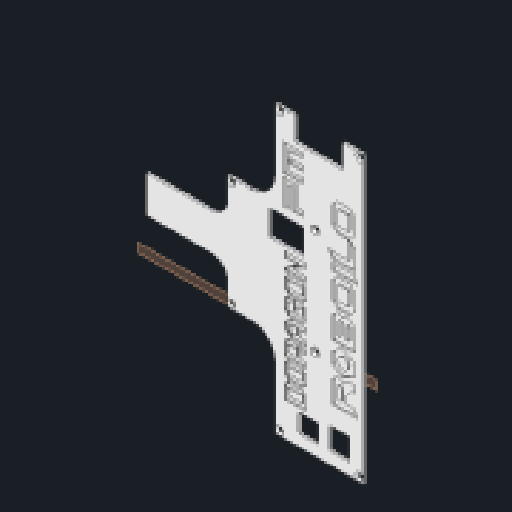
# Autodesk Inventor part: ceil
Saved by Autodesk Inventor 2023 (Build 270158000, 158)
## iProperties
Created: 2024-05-26
Part Number: ceil
Material: ABS Plastic
Document SubType Name: Modeling
Designer: szymo
Density: 1.06 g/cm^3
Appearance: Smooth - White
Mass: 19.1386 g
Surface Area: 254.518 cm^2
Volume: 18.0553 cm^3
TOTAL MASS: 0.0
Author: szymo
Autodesk Inventor part; units mm, degrees
ref_plane "YZ Plane" through (0, 0, 0) normal (1, 0, 0) x (0, 1, 0)
ref_plane "XZ Plane" through (0, 0, 0) normal (0, 1, 0) x (-1, 0, 0)
ref_plane "XY Plane" through (0, 0, 0) normal (0, 0, 1) x (1, 0, 0)
ref_plane "Work Plane1" through (-50.5, 0, 0) normal (0, 0, 1) x (1, 0, 0)
sketch "Sketch3" plane through (-50.5, 0, 0) normal (0, 0, 1) x (1, 0, 0)
  line L0 (0, 0) -> (135.5648, 0) projected
  line L1 (135.5648, 0) -> (135.5648, 5) projected
  line L2 (0, 5) -> (135.5648, 5) projected
  line L3 (0, 0) -> (0, 5) projected
  line L4 (0, 24) -> (50.5, 24) projected
  line L5 (0, 47) -> (50.5, 47) projected
  line L6 (0, 71) -> (135.5648, 71) projected
  line L7 (0, 71) -> (0, 66) projected
  line L8 (0, 66) -> (135.5648, 66) projected
  line L9 (135.5648, 71) -> (135.5648, 66) projected
  arc A0 (130.5648, 120.5) -> (131.5648, 119.5) centre (131.5648, 120.5) ccw projected
  line L10 (131.5648, 119.5) -> (134.5648, 119.5) projected
  arc A1 (134.5648, 119.5) -> (135.5648, 120.5) centre (134.5648, 120.5) ccw projected
  line L11 (135.5648, 124.5) -> (135.5648, 120.5) projected
  line L12 (135.5648, 124.5) -> (51.5, 124.5) projected
  line L13 (51.5, 123.5) -> (80.5, 123.5) projected
  line L14 (80.5, 123.5) -> (80.5, 120.5) projected
  arc A2 (80.5, 120.5) -> (81.5, 119.5) centre (81.5, 120.5) ccw projected
  line L15 (81.5, 119.5) -> (84.5, 119.5) projected
  arc A3 (84.5, 119.5) -> (85.5, 120.5) centre (84.5, 120.5) ccw projected
  line L16 (85.5, 123.5) -> (85.5, 120.5) projected
  line L17 (85.5, 123.5) -> (130.5648, 123.5) projected
  line L18 (130.5648, 123.5) -> (130.5648, 120.5) projected
  circle A4 centre (133.0648, 122) radius 1.75 projected
  circle A5 centre (83, 122) radius 1.75 projected
  line L19 (120.8148, 112) -> (120.8148, 123) projected
  line L20 (120.8148, 123) -> (94.8148, 123) projected
  line L21 (94.8148, 123) -> (94.8148, 112) projected
  line L22 (94.8148, 112) -> (120.8148, 112) projected
  arc A6 (131.5648, -48.5) -> (130.5648, -49.5) centre (131.5648, -49.5) ccw projected
  line L23 (130.5648, -52.5) -> (130.5648, -49.5) projected
  line L24 (85.5, -52.5) -> (130.5648, -52.5) projected
  line L25 (85.5, -52.5) -> (85.5, -49.5) projected
  arc A7 (85.5, -49.5) -> (84.5, -48.5) centre (84.5, -49.5) ccw projected
  line L26 (81.5, -48.5) -> (84.5, -48.5) projected
  arc A8 (81.5, -48.5) -> (80.5, -49.5) centre (81.5, -49.5) ccw projected
  line L27 (80.5, -52.5) -> (80.5, -49.5) projected
  line L28 (51.5, -52.5) -> (80.5, -52.5) projected
  line L29 (135.5648, -53.5) -> (51.5, -53.5) projected
  line L30 (135.5648, -53.5) -> (135.5648, -49.5) projected
  arc A9 (135.5648, -49.5) -> (134.5648, -48.5) centre (134.5648, -49.5) ccw projected
  line L31 (131.5648, -48.5) -> (134.5648, -48.5) projected
  circle A10 centre (133.0648, -51) radius 1.75 projected
  circle A11 centre (83, -51) radius 1.75 projected
  line L32 (95.5648, -45.8) -> (95.5648, -35.2) projected
  line L33 (106.8648, -35.2) -> (95.5648, -35.2) projected
  line L34 (106.8648, -35.2) -> (106.8648, -45.8) projected
  line L35 (95.5648, -45.8) -> (106.8648, -45.8) projected
  circle A12 centre (90.4898, -49.075) radius 1.675 projected
  circle A13 centre (124.5398, -49.075) radius 1.675 projected
  line L36 (126.3648, -33.5) -> (126.3648, -45.5) projected
  line L37 (126.3648, -45.5) -> (114.7648, -45.5) projected
  line L38 (114.7648, -45.5) -> (114.7648, -33.5) projected
  line L39 (114.7648, -33.5) -> (86.8648, -33.5) projected
  line L40 (86.8648, -33.5) -> (86.8648, -52.5) projected
  line L41 (86.8648, -52.5) -> (128.0648, -52.5) projected
  line L42 (128.0648, -52.5) -> (128.0648, -33.5) projected
  line L43 (128.0648, -33.5) -> (126.3648, -33.5) projected
  line L44 (126.3648, -32.7) -> (114.7648, -32.7) projected
  line L45 (114.7648, -32.7) -> (114.7648, -45.5) projected
  line L46 (114.7648, -45.5) -> (126.3648, -45.5) projected
  line L47 (126.3648, -45.5) -> (126.3648, -32.7) projected
  line L48 (80.5, -53.5) -> (135.5648, -53.5)
  line L49 (135.5648, -53.5) -> (135.5648, 124.5)
  line L50 (135.5648, 124.5) -> (80.5, 124.5)
  line L51 (80.5, 124.5) -> (80.5, -53.5)
  line L52 (0, 24) -> (80.5, 24)
  line L53 (80.5, 24) -> (80.5, 47)
  line L54 (80.5, 47) -> (0, 47)
  line L55 (0, 47) -> (0, 24)
  line L56 (80.5, 24) -> (50.5, 24)
  line L57 (50.5, 24) -> (50.5, 0)
  line L58 (50.5, 0) -> (80.5, 0)
  line L59 (80.5, 0) -> (80.5, 24)
  line L60 (50.5, 47) -> (80.5, 47)
  line L61 (80.5, 47) -> (80.5, 71)
  line L62 (80.5, 71) -> (50.5, 71)
  line L63 (50.5, 71) -> (50.5, 47)
  arc A14 (97.9124, 51.3) -> (98.0124, 51.4) centre (97.9124, 51.4) ccw projected
  line L64 (77.4124, 51.3) -> (97.9124, 51.3) projected
  arc A15 (77.3124, 51.4) -> (77.4124, 51.3) centre (77.4124, 51.4) ccw projected
  line L65 (77.3124, 65.9) -> (77.3124, 51.4) projected
  arc A16 (77.4124, 66) -> (77.3124, 65.9) centre (77.4124, 65.9) ccw projected
  line L66 (97.9124, 66) -> (77.4124, 66) projected
  arc A17 (98.0124, 65.9) -> (97.9124, 66) centre (97.9124, 65.9) ccw projected
  line L67 (98.0124, 51.4) -> (98.0124, 65.9) projected
  line L68 (96.2124, 64.1) -> (96.2124, 53.2) projected
  arc A18 (96.2124, 64.1) -> (95.9124, 64.4) centre (95.9124, 64.1) ccw projected
  line L69 (95.9124, 64.4) -> (95.8124, 64.4) projected
  line L70 (95.8124, 64.4) -> (95.3509, 64.95) projected
  line L71 (95.3509, 64.95) -> (94.9739, 64.95) projected
  line L72 (94.9739, 64.95) -> (94.5124, 64.4) projected
  line L73 (94.5124, 64.4) -> (90.8124, 64.4) projected
  line L74 (90.8124, 64.4) -> (90.8124, 64.75) projected
  line L75 (90.8124, 64.75) -> (89.5124, 64.75) projected
  line L76 (89.5124, 64.4) -> (89.5124, 64.75) projected
  line L77 (89.5124, 64.4) -> (85.8124, 64.4) projected
  line L78 (85.8124, 64.4) -> (85.8124, 64.75) projected
  line L79 (85.8124, 64.75) -> (84.5124, 64.75) projected
  line L80 (84.5124, 64.4) -> (84.5124, 64.75) projected
  line L81 (84.5124, 64.4) -> (80.8124, 64.4) projected
  line L82 (80.8124, 64.4) -> (80.3509, 64.95) projected
  line L83 (80.3509, 64.95) -> (79.9739, 64.95) projected
  line L84 (79.9739, 64.95) -> (79.5124, 64.4) projected
  line L85 (79.5124, 64.4) -> (79.4124, 64.4) projected
  arc A19 (79.4124, 64.4) -> (79.1124, 64.1) centre (79.4124, 64.1) ccw projected
  line L86 (79.1124, 64.1) -> (79.1124, 53.2) projected
  arc A20 (79.1124, 53.2) -> (79.4124, 52.9) centre (79.4124, 53.2) ccw projected
  line L87 (79.4124, 52.9) -> (79.5124, 52.9) projected
  line L88 (79.5124, 52.9) -> (79.9739, 52.35) projected
  line L89 (80.3509, 52.35) -> (79.9739, 52.35) projected
  line L90 (80.3509, 52.35) -> (80.8124, 52.9) projected
  line L91 (80.8124, 52.9) -> (84.5124, 52.9) projected
  line L92 (84.5124, 52.9) -> (84.5124, 52.55) projected
  line L93 (85.8124, 52.55) -> (84.5124, 52.55) projected
  line L94 (85.8124, 52.9) -> (85.8124, 52.55) projected
  line L95 (85.8124, 52.9) -> (89.5124, 52.9) projected
  line L96 (89.5124, 52.9) -> (89.5124, 52.55) projected
  line L97 (90.8124, 52.55) -> (89.5124, 52.55) projected
  line L98 (90.8124, 52.9) -> (90.8124, 52.55) projected
  line L99 (90.8124, 52.9) -> (94.5124, 52.9) projected
  line L100 (94.5124, 52.9) -> (94.9739, 52.35) projected
  line L101 (95.3509, 52.35) -> (94.9739, 52.35) projected
  line L102 (95.3509, 52.35) -> (95.8124, 52.9) projected
  line L103 (95.8124, 52.9) -> (95.9124, 52.9) projected
  arc A21 (95.9124, 52.9) -> (96.2124, 53.2) centre (95.9124, 53.2) ccw projected
  line L104 (78.1624, 55.75) -> (78.8624, 55.75) projected
  line L105 (78.8624, 55.75) -> (78.8624, 61.55) projected
  line L106 (78.1624, 61.55) -> (78.8624, 61.55) projected
  line L107 (78.1624, 61.55) -> (78.1624, 55.75) projected
  line L108 (97.1624, 61.55) -> (97.1624, 55.75) projected
  line L109 (96.4624, 61.55) -> (97.1624, 61.55) projected
  line L110 (96.4624, 55.75) -> (96.4624, 61.55) projected
  line L111 (96.4624, 55.75) -> (97.1624, 55.75) projected
  arc A22 (76.8124, 51.4) -> (77.4124, 50.8) centre (77.4124, 51.4) ccw
  line L112 (77.4124, 50.8) -> (97.9124, 50.8)
  arc A23 (97.9124, 50.8) -> (98.5124, 51.4) centre (97.9124, 51.4) ccw
  line L113 (98.5124, 51.4) -> (98.5124, 65.9)
  arc A24 (98.5124, 65.9) -> (97.9124, 66.5) centre (97.9124, 65.9) ccw
  line L114 (97.9124, 66.5) -> (77.4124, 66.5)
  arc A25 (77.4124, 66.5) -> (76.8124, 65.9) centre (77.4124, 65.9) ccw
  line L115 (76.8124, 65.9) -> (76.8124, 51.4)
  line L116 (95.0648, -34.7) -> (95.0648, -46.3)
  line L117 (95.0648, -46.3) -> (107.3648, -46.3)
  line L118 (107.3648, -46.3) -> (107.3648, -34.7)
  line L119 (107.3648, -34.7) -> (95.0648, -34.7)
  line L120 (114.2648, -45.5) -> (114.2648, -32.2)
  line L121 (114.2648, -32.2) -> (126.8648, -32.2)
  line L122 (126.8648, -32.2) -> (126.8648, -45.5)
  line L123 (126.3648, -46) -> (114.7648, -46)
  line L124 (92.8148, 110) -> (92.8148, 125)
  line L125 (92.8148, 125) -> (122.8148, 125)
  line L126 (122.8148, 125) -> (122.8148, 110)
  line L127 (122.8148, 110) -> (92.8148, 110)
  line L128 (114.2648, -45.5) -> (114.2648, -46)
  line L129 (114.2648, -46) -> (114.7648, -46)
  line L130 (126.3648, -46) -> (126.8648, -46)
  line L131 (126.8648, -46) -> (126.8648, -45.5)
  line L132 (51.5, -53.5) -> (51.5, -52.5) projected
  line L133 (51.5, 124.5) -> (51.5, 123.5) projected
  circle A26 centre (105.3205, 68.5) radius 1.75 projected
  circle A27 centre (53, 68.5) radius 1.75 projected
  line L134 (0, 47) -> (0, 42.5) projected
  line L135 (0, 42.5) -> (50.5, 42.5) projected
  line L136 (50.5, 47) -> (50.5, 42.5) projected
  line L137 (50.5, 24) -> (50.5, 28.5) projected
  line L138 (0, 28.5) -> (50.5, 28.5) projected
  line L139 (0, 24) -> (0, 28.5) projected
  circle A28 centre (105.3205, 2.5) radius 1.75 projected
  circle A29 centre (53, 2.5) radius 1.75 projected
  point P0 (122.8148, 124.5)
  point P1 (92.8148, 124.5)
  point P2 (80.5, 0)
  point P3 (0, 44)
  point P4 (50.5, 44)
  point P5 (122.8148, 124.5)
  point P6 (122.8148, 123.5)
  point P7 (92.8148, 123.5)
  point P8 (92.8148, 124.5)
  point P9 (50.5, 66)
  point P10 (50.5, 5)
  point P11 (80.5, 66)
  point P12 (80.5, 5)
  point P13 (50.5, 27)
  point P14 (0, 27)
  dimension "d16" = 0.5
  dimension "d17" = 0.5
  dimension "d18" = 0.5
  dimension "d19" = 0.5
  dimension "d20" = 2
  constraints: 72 end point, 9 parallel, 8 point on circle, 6 perpendicular, 5 point on line, 4 centre point, 4 horizontal, 2 collinear, 1 vertical, 15 other
  measures "d16" distance between parallel lines of L65 L115
  measures "d17" distance between parallel lines of L32 L116
  measures "d18" distance between parallel lines of L45 L120
  measures "d19" distance between parallel lines of L37 L123
  measures "d20" distance between parallel lines of L21 L124
extrude "Extrusion2" add sketch "Sketch3" along normal blind 1.5 contours L57 L2 L51 L0 | L51 L2 L1 L0 | L0 L49 A9 L31 A6 L23 L24 L42 L43 L122 L121 L120 L39 L40 L25 A7 L26 A8 L51 | L57 L52 L51 L2 | A8 L26 A7 L25 L24 L23 A6 L31 A9 L30 L29 L51 L27 | L51 L112 A23 L113 A24 L8 L49 L2 | L137 L138 L55 L135 L136 L54 L51 L52 | L4 L55 L138 L137 | L8 A24 L114 L51 L6 L9 | L54 L63 L8 A25 L115 A22 L112 L51 | L6 L51 A2 L15 A3 L16 L17 L124 L127 L126 L18 A0 L10 A1 L49 | L136 L135 L55 L5 | L51 L114 A25 L8 L63 L6 | A1 L10 A0 L18 L17 L126 L12 L11 | L14 L51 L12 L124 L17 L16 A3 L15 A2 | L40 L39 L120 L128 L129 L123 L130 L131 L122 L43 L42 L24 | A4 | A5 | A10 | A11 | A12 | A13 | A26 | A27 | A28 | A29
fillet "Fillet2" radius 1 10 edges at (44.5648, -46.3, 0.75) (44.5648, -34.7, 0.75) (56.8648, -34.7, 0.75) (56.8648, -46.3, 0.75) (63.7648, -46, 0.75) (63.7648, -32.2, 0.75) (76.3648, -32.2, 0.75) (76.3648, -46, 0.75) (42.3148, 110, 0.75) (72.3148, 110, 0.75)
fillet "Fillet3" radius 15 2 edges at (30, 0, 0.75) (30, 71, 0.75)
sketch "Sketch4" plane through (-50.5, 0, 1.5) normal (0, 0, 1) x (1, 0, 0)
  arc A0 (131.5648, -48.5) -> (130.5648, -49.5) centre (131.5648, -49.5) ccw projected
  line L0 (130.5648, -52.5) -> (130.5648, -49.5) projected
  line L1 (85.5, -52.5) -> (130.5648, -52.5) projected
  line L2 (85.5, -52.5) -> (85.5, -49.5) projected
  arc A1 (85.5, -49.5) -> (84.5, -48.5) centre (84.5, -49.5) ccw projected
  line L3 (81.5, -48.5) -> (84.5, -48.5) projected
  arc A2 (81.5, -48.5) -> (80.5, -49.5) centre (81.5, -49.5) ccw projected
  line L4 (80.5, -52.5) -> (80.5, -49.5) projected
  line L5 (51.5, -52.5) -> (80.5, -52.5) projected
  line L6 (135.5648, -53.5) -> (51.5, -53.5) projected
  line L7 (135.5648, -53.5) -> (135.5648, -49.5) projected
  arc A3 (135.5648, -49.5) -> (134.5648, -48.5) centre (134.5648, -49.5) ccw projected
  line L8 (131.5648, -48.5) -> (134.5648, -48.5) projected
  circle A4 centre (133.0648, -51) radius 1.75 projected
  circle A5 centre (83, -51) radius 1.75 projected
  arc A6 (130.5648, 120.5) -> (131.5648, 119.5) centre (131.5648, 120.5) ccw projected
  line L9 (131.5648, 119.5) -> (134.5648, 119.5) projected
  arc A7 (134.5648, 119.5) -> (135.5648, 120.5) centre (134.5648, 120.5) ccw projected
  line L10 (135.5648, 124.5) -> (135.5648, 120.5) projected
  line L11 (135.5648, 124.5) -> (51.5, 124.5) projected
  line L12 (51.5, 123.5) -> (80.5, 123.5) projected
  line L13 (80.5, 123.5) -> (80.5, 120.5) projected
  arc A8 (80.5, 120.5) -> (81.5, 119.5) centre (81.5, 120.5) ccw projected
  line L14 (81.5, 119.5) -> (84.5, 119.5) projected
  arc A9 (84.5, 119.5) -> (85.5, 120.5) centre (84.5, 120.5) ccw projected
  line L15 (85.5, 123.5) -> (85.5, 120.5) projected
  line L16 (85.5, 123.5) -> (130.5648, 123.5) projected
  line L17 (130.5648, 123.5) -> (130.5648, 120.5) projected
  circle A10 centre (133.0648, 122) radius 1.75 projected
  circle A11 centre (83, 122) radius 1.75 projected
  line L18 (0, 71) -> (135.5648, 71) projected
  line L19 (0, 71) -> (0, 66) projected
  line L20 (0, 66) -> (135.5648, 66) projected
  line L21 (135.5648, 71) -> (135.5648, 66) projected
  line L22 (0, 0) -> (135.5648, 0) projected
  line L23 (135.5648, 0) -> (135.5648, 5) projected
  line L24 (0, 5) -> (135.5648, 5) projected
  line L25 (0, 0) -> (0, 5) projected
  line L26 (0, 24) -> (50.5, 24) projected
  line L27 (0, 47) -> (50.5, 47) projected
  line L28 (51.5, 124.5) -> (51.5, 123.5) projected
  line L29 (51.5, -53.5) -> (51.5, -52.5) projected
  circle A12 centre (105.3205, 68.5) radius 1.75 projected
  circle A13 centre (53, 68.5) radius 1.75 projected
  line L30 (0, 47) -> (0, 42.5) projected
  line L31 (0, 42.5) -> (50.5, 42.5) projected
  line L32 (50.5, 47) -> (50.5, 42.5) projected
  line L33 (50.5, 24) -> (50.5, 28.5) projected
  line L34 (0, 28.5) -> (50.5, 28.5) projected
  line L35 (0, 24) -> (0, 28.5) projected
  circle A14 centre (105.3205, 2.5) radius 1.75 projected
  circle A15 centre (53, 2.5) radius 1.75 projected
  point P0 (50.5, 0)
  point P1 (0, 44)
  point P2 (50.5, 44)
  point P3 (50.5, 27)
  point P4 (0, 27)
  constraints: 8 coincident
hole "Hole2" at (32.5, -51, 1.5) at (82.5648, -51, 1.5) at (82.5648, 122, 1.5) at (32.5, 122, 1.5) at (54.8205, 68.5, 1.5) at (54.8205, 2.5, 1.5) at (2.5, 2.5, 1.5) at (2.5, 68.5, 1.5) direction (0, 0, -1) diameter 2.9 end through all countersink diameter 5.5 countersink angle 90 clearance for "Countersunk Flat Head Screw ISO 2009/7046" size "M2.5" standard "ISO"
fillet "Fillet4" radius 10 2 edges at (0, 24, 0.75) (0, 47, 0.75)
sketch "Sketch5" plane through (-50.5, 0, 1.5) normal (0, 0, 1) x (1, 0, 0)
  arc A0 (54.1456, 0) -> (50.5, 3.6456) centre (53, 2.5) ccw projected
  line L0 (54.1456, 0) -> (65.5, 0) projected
  arc A1 (80.5, -15) -> (65.5, 0) centre (65.5, -15) ccw projected
  line L1 (80.5, -15) -> (80.5, -49.8544) projected
  arc A2 (84.1456, -53.5) -> (80.5, -49.8544) centre (83, -51) ccw projected
  line L2 (84.1456, -53.5) -> (131.9191, -53.5) projected
  arc A3 (135.5648, -49.8544) -> (131.9191, -53.5) centre (133.0648, -51) ccw projected
  line L3 (135.5648, -49.8544) -> (135.5648, 120.8544) projected
  arc A4 (131.9191, 124.5) -> (135.5648, 120.8544) centre (133.0648, 122) ccw projected
  line L4 (131.9191, 124.5) -> (122.8148, 124.5) projected
  line L5 (122.8148, 124.5) -> (122.8148, 111) projected
  arc A5 (121.8148, 110) -> (122.8148, 111) centre (121.8148, 111) ccw projected
  line L6 (121.8148, 110) -> (93.8148, 110) projected
  arc A6 (92.8148, 111) -> (93.8148, 110) centre (93.8148, 111) ccw projected
  line L7 (92.8148, 111) -> (92.8148, 124.5) projected
  line L8 (92.8148, 124.5) -> (84.1456, 124.5) projected
  arc A7 (80.5, 120.8544) -> (84.1456, 124.5) centre (83, 122) ccw projected
  line L9 (80.5, 120.8544) -> (80.5, 86) projected
  arc A8 (65.5, 71) -> (80.5, 86) centre (65.5, 86) ccw projected
  line L10 (65.5, 71) -> (54.1456, 71) projected
  arc A9 (50.5, 67.3544) -> (54.1456, 71) centre (53, 68.5) ccw projected
  line L11 (50.5, 67.3544) -> (50.5, 57) projected
  arc A10 (40.5, 47) -> (50.5, 57) centre (40.5, 57) ccw projected
  line L12 (40.5, 47) -> (0, 47) projected
  line L13 (0, 47) -> (0, 24) projected
  line L14 (0, 24) -> (40.5, 24) projected
  arc A11 (50.5, 14) -> (40.5, 24) centre (40.5, 14) ccw projected
  line L15 (50.5, 14) -> (50.5, 3.6456) projected
  circle A12 centre (105.3205, 68.5) radius 2.75 projected
  circle A13 centre (105.3205, 2.5) radius 2.75 projected
  line L16 (77.4124, 66.5) -> (97.9124, 66.5) projected
  arc A14 (98.5124, 65.9) -> (97.9124, 66.5) centre (97.9124, 65.9) ccw projected
  line L17 (98.5124, 65.9) -> (98.5124, 51.4) projected
  arc A15 (97.9124, 50.8) -> (98.5124, 51.4) centre (97.9124, 51.4) ccw projected
  line L18 (97.9124, 50.8) -> (77.4124, 50.8) projected
  arc A16 (76.8124, 51.4) -> (77.4124, 50.8) centre (77.4124, 51.4) ccw projected
  line L19 (76.8124, 51.4) -> (76.8124, 65.9) projected
  arc A17 (77.4124, 66.5) -> (76.8124, 65.9) centre (77.4124, 65.9) ccw projected
  line L20 (114.2648, -45) -> (114.2648, -33.2) projected
  arc A18 (115.2648, -32.2) -> (114.2648, -33.2) centre (115.2648, -33.2) ccw projected
  line L21 (115.2648, -32.2) -> (125.8648, -32.2) projected
  arc A19 (126.8648, -33.2) -> (125.8648, -32.2) centre (125.8648, -33.2) ccw projected
  line L22 (126.8648, -33.2) -> (126.8648, -45) projected
  arc A20 (125.8648, -46) -> (126.8648, -45) centre (125.8648, -45) ccw projected
  line L23 (125.8648, -46) -> (115.2648, -46) projected
  arc A21 (114.2648, -45) -> (115.2648, -46) centre (115.2648, -45) ccw projected
  line L24 (96.0648, -34.7) -> (106.3648, -34.7) projected
  arc A22 (107.3648, -35.7) -> (106.3648, -34.7) centre (106.3648, -35.7) ccw projected
  line L25 (107.3648, -35.7) -> (107.3648, -45.3) projected
  arc A23 (106.3648, -46.3) -> (107.3648, -45.3) centre (106.3648, -45.3) ccw projected
  line L26 (106.3648, -46.3) -> (96.0648, -46.3) projected
  arc A24 (95.0648, -45.3) -> (96.0648, -46.3) centre (96.0648, -45.3) ccw projected
  line L27 (95.0648, -45.3) -> (95.0648, -35.7) projected
  arc A25 (96.0648, -34.7) -> (95.0648, -35.7) centre (96.0648, -35.7) ccw projected
  line L28 (105.3205, -31.7) -> (105.3205, 48.8) construction
  line L29 (105.3205, 48.8) -> (80.5, 48.8) construction
  line L30 (80.5, 48.8) -> (80.5, -31.7) construction
  line L31 (80.5, -31.7) -> (105.3205, -31.7) construction
  line L32 (116.1651, 28.6458) -> (116.1651, 14.5717) projected
  line L33 (125.2148, -10.52) -> (128.2141, -7.4431) projected
  line L34 (128.2141, -7.4431) -> (129.5648, -7.4431) projected
  line L35 (129.5648, -7.4431) -> (129.5648, -3.1151) projected
  line L36 (129.5648, -3.1151) -> (125.5551, -3.1151) projected
  line L37 (125.5551, -3.1151) -> (123.3584, -5.3021) projected
  line L38 (123.3584, -5.3021) -> (120.3535, -3.0659) projected
  line L39 (120.3535, -3.0659) -> (116.1651, -6.1782) projected
  line L40 (116.1651, -6.1782) -> (116.1651, -20.0711) projected
  line L41 (116.1651, -20.0711) -> (131.9602, -20.0711) projected
  line L42 (131.9602, -20.0711) -> (129.4807, -15.7431) projected
  line L43 (129.4807, -15.7431) -> (125.2148, -15.7431) projected
  line L44 (125.2148, -15.7431) -> (125.2148, -10.52) projected
  line L45 (120.6271, -7.6036) -> (121.8612, -8.5098) projected
  line L46 (121.8612, -8.5098) -> (121.8612, -15.7431) projected
  line L47 (121.8612, -15.7431) -> (119.4584, -15.7431) projected
  line L48 (119.4584, -15.7431) -> (119.4584, -8.4973) projected
  line L49 (119.4584, -8.4973) -> (120.6271, -7.6036) projected
  line L50 (129.5648, 1.4254) -> (129.5648, 9.1617) projected
  line L51 (129.5648, 9.1617) -> (122.8649, 13.0299) projected
  line L52 (122.8649, 13.0299) -> (116.1651, 9.1617) projected
  line L53 (116.1651, 9.1617) -> (116.1651, 1.4254) projected
  line L54 (116.1651, 1.4254) -> (122.8649, -2.4427) projected
  line L55 (122.8649, -2.4427) -> (129.5648, 1.4254) projected
  circle A26 centre (122.8649, 5.2936) radius 3.3 projected
  line L56 (129.5848, 14.5717) -> (129.5848, 28.6458) projected
  line L57 (129.5848, 28.6458) -> (125.3867, 31.747) projected
  line L58 (125.3867, 31.747) -> (122.875, 29.8983) projected
  line L59 (122.875, 29.8983) -> (120.3632, 31.747) projected
  line L60 (120.3632, 31.747) -> (116.1651, 28.6458) projected
  line L61 (116.1651, 28.6458) -> (116.1651, 14.5717) projected
  line L62 (116.1651, 14.5717) -> (129.5848, 14.5717) projected
  line L63 (121.3489, 26.1486) -> (121.3489, 18.8997) projected
  line L64 (121.3489, 18.8997) -> (119.4785, 18.8997) projected
  line L65 (119.4785, 18.8997) -> (119.4785, 26.1539) projected
  line L66 (119.4785, 26.1539) -> (120.3691, 26.9374) projected
  line L67 (120.3691, 26.9374) -> (121.3489, 26.1486) projected
  line L68 (124.4011, 18.8997) -> (124.4011, 26.1486) projected
  line L69 (124.4011, 26.1486) -> (125.3808, 26.9374) projected
  line L70 (125.3808, 26.9374) -> (126.2715, 26.1539) projected
  line L71 (126.2715, 26.1539) -> (126.2715, 18.8997) projected
  line L72 (126.2715, 18.8997) -> (124.4011, 18.8997) projected
  line L73 (126.494, 33.3579) -> (129.5648, 36.4286) projected
  line L74 (129.5648, 36.4286) -> (129.5648, 47.4441) projected
  line L75 (129.5648, 47.4441) -> (126.494, 50.5148) projected
  line L76 (126.494, 50.5148) -> (119.2358, 50.5148) projected
  line L77 (119.2358, 50.5148) -> (116.1651, 47.4441) projected
  line L78 (116.1651, 47.4441) -> (116.1651, 36.4286) projected
  line L79 (116.1651, 36.4286) -> (119.2358, 33.3579) projected
  line L80 (119.2358, 33.3579) -> (126.494, 33.3579) projected
  line L81 (126.2715, 37.686) -> (119.4584, 37.686) projected
  line L82 (119.4584, 37.686) -> (119.4584, 46.1868) projected
  line L83 (119.4584, 46.1868) -> (126.2715, 46.1868) projected
  line L84 (126.2715, 46.1868) -> (126.2715, 37.686) projected
  line L85 (131.9586, 52.2145) -> (129.5013, 56.5425) projected
  line L86 (129.5013, 56.5425) -> (116.1651, 56.5425) projected
  line L87 (116.1651, 56.5425) -> (116.1651, 52.2145) projected
  line L88 (116.1651, 52.2145) -> (131.9586, 52.2145) projected
  line L89 (129.5648, 88.0003) -> (126.494, 91.071) projected
  line L90 (126.494, 91.071) -> (119.2358, 91.071) projected
  line L91 (119.2358, 91.071) -> (116.1651, 88.0003) projected
  line L92 (116.1651, 88.0003) -> (116.1651, 76.9848) projected
  line L93 (116.1651, 76.9848) -> (119.2358, 73.9141) projected
  line L94 (119.2358, 73.9141) -> (126.2715, 73.9141) projected
  line L95 (126.2715, 73.9141) -> (126.2715, 62.7008) projected
  line L96 (126.2715, 62.7008) -> (113.738, 62.7008) projected
  line L97 (113.738, 62.7008) -> (116.2396, 58.3727) projected
  line L98 (116.2396, 58.3727) -> (129.5848, 58.3727) projected
  line L99 (129.5848, 58.3727) -> (129.5848, 70.8415) projected
  line L100 (129.5848, 70.8415) -> (126.5032, 73.9232) projected
  line L101 (126.5032, 73.9232) -> (129.5648, 76.9848) projected
  line L102 (129.5648, 76.9848) -> (129.5648, 88.0003) projected
  line L103 (126.2715, 78.2421) -> (119.4584, 78.2421) projected
  line L104 (119.4584, 78.2421) -> (119.4584, 86.743) projected
  line L105 (119.4584, 86.743) -> (126.2715, 86.743) projected
  line L106 (126.2715, 86.743) -> (126.2715, 78.2421) projected
  line L107 (91.5024, 71.975) -> (97.5262, 71.975) projected
  line L108 (97.5262, 71.975) -> (97.5262, 74.9242) projected
  line L109 (97.5262, 74.9242) -> (94.45, 74.9242) projected
  line L110 (94.45, 74.9242) -> (94.45, 87.525) projected
  line L111 (94.45, 87.525) -> (85.5, 87.525) projected
  line L112 (85.5, 87.525) -> (85.5, 71.975) projected
  line L113 (85.5, 71.975) -> (88.675, 71.975) projected
  line L114 (88.675, 71.975) -> (88.675, 84.4887) projected
  line L115 (88.675, 84.4887) -> (91.5024, 84.4887) projected
  line L116 (91.5024, 84.4887) -> (91.5024, 71.975) projected
  line L117 (85.5, 106.5) -> (85.5, 89.825) projected
  line L118 (85.5, 89.825) -> (97.6, 89.825) projected
  line L119 (97.6, 89.825) -> (97.6, 92.775) projected
  line L120 (97.6, 92.775) -> (88.6, 92.775) projected
  line L121 (88.6, 92.775) -> (88.6, 103.4705) projected
  line L122 (88.6, 103.4705) -> (97.5254, 103.4705) projected
  line L123 (97.5254, 103.4705) -> (97.5254, 106.5) projected
  line L124 (97.5254, 106.5) -> (85.5, 106.5) projected
  line L125 (89.7, 99.675) -> (89.7, 96.575) projected
  line L126 (89.7, 96.575) -> (97.6, 96.575) projected
  line L127 (97.6, 96.575) -> (97.6, 99.675) projected
  line L128 (97.6, 99.675) -> (89.7, 99.675) projected
  circle A27 centre (105.3205, 2.5) radius 2.75 projected
  line L129 (99.4102, -32.075) -> (86.4102, -32.075)
  line L130 (86.4102, -32.075) -> (86.4102, -23.2821)
  line L131 (86.4102, -23.2821) -> (88.2317, -23.2821)
  line L132 (88.2317, -23.2821) -> (88.2317, -21.8607)
  line L133 (88.2317, -21.8607) -> (97.5888, -21.8607)
  line L134 (97.5888, -21.8607) -> (97.5888, -23.2821)
  line L135 (97.5888, -23.2821) -> (99.4102, -23.2821)
  line L136 (99.4102, -23.2821) -> (99.4102, -32.075)
  line L137 (97.3317, -24.9679) -> (88.4888, -24.9679)
  line L138 (88.4888, -24.9679) -> (88.4888, -28.9679)
  line L139 (88.4888, -28.9679) -> (97.3317, -28.9679)
  line L140 (97.3317, -28.9679) -> (97.3317, -24.9679)
  line L141 (99.4102, -19.0464) -> (97.5888, -19.0464)
  line L142 (97.5888, -19.0464) -> (97.5888, -20.4679)
  line L143 (97.5888, -20.4679) -> (88.2317, -20.4679)
  line L144 (88.2317, -20.4679) -> (88.2317, -19.0464)
  line L145 (88.2317, -19.0464) -> (86.4102, -19.0464)
  line L146 (86.4102, -19.0464) -> (86.4102, -11.675)
  line L147 (86.4102, -11.675) -> (88.2317, -11.675)
  line L148 (88.2317, -11.675) -> (88.2317, -10.2536)
  line L149 (88.2317, -10.2536) -> (97.5888, -10.2536)
  line L150 (97.5888, -10.2536) -> (97.5888, -11.675)
  line L151 (97.5888, -11.675) -> (99.4102, -11.675)
  line L152 (99.4102, -11.675) -> (99.4102, -19.0464)
  line L153 (97.3317, -13.3607) -> (88.4888, -13.3607)
  line L154 (88.4888, -13.3607) -> (88.4888, -17.3607)
  line L155 (88.4888, -17.3607) -> (97.3317, -17.3607)
  line L156 (97.3317, -17.3607) -> (97.3317, -13.3607)
  line L157 (99.4102, -8.8607) -> (86.4102, -8.8607)
  line L158 (86.4102, -8.8607) -> (86.4102, -0.0679)
  line L159 (86.4102, -0.0679) -> (88.2317, -0.0679)
  line L160 (88.2317, -0.0679) -> (88.2317, 1.3536)
  line L161 (88.2317, 1.3536) -> (93.9531, 1.3536)
  line L162 (93.9531, 1.3536) -> (93.9531, -0.0679)
  line L163 (93.9531, -0.0679) -> (95.5102, -0.0679)
  line L164 (95.5102, -0.0679) -> (95.5102, 1.3536)
  line L165 (95.5102, 1.3536) -> (99.4102, 1.3536)
  line L166 (99.4102, 1.3536) -> (99.4102, -1.7536)
  line L167 (99.4102, -1.7536) -> (95.7674, -1.7536)
  line L168 (95.7674, -1.7536) -> (95.7674, -5.7536)
  line L169 (95.7674, -5.7536) -> (99.4102, -5.7536)
  line L170 (99.4102, -5.7536) -> (99.4102, -8.8607)
  line L171 (93.6959, -1.7536) -> (88.4888, -1.7536)
  line L172 (88.4888, -1.7536) -> (88.4888, -5.7536)
  line L173 (88.4888, -5.7536) -> (93.6959, -5.7536)
  line L174 (93.6959, -5.7536) -> (93.6959, -1.7536)
  line L175 (99.4102, 2.7464) -> (90.0531, 2.7464)
  line L176 (90.0531, 2.7464) -> (90.0531, 4.1679)
  line L177 (90.0531, 4.1679) -> (88.2317, 4.1679)
  line L178 (88.2317, 4.1679) -> (88.2317, 5.5893)
  line L179 (88.2317, 5.5893) -> (86.4102, 5.5893)
  line L180 (86.4102, 5.5893) -> (86.4102, 10.1179)
  line L181 (86.4102, 10.1179) -> (88.2317, 10.1179)
  line L182 (88.2317, 10.1179) -> (88.2317, 11.5393)
  line L183 (88.2317, 11.5393) -> (90.0531, 11.5393)
  line L184 (90.0531, 11.5393) -> (90.0531, 12.9607)
  line L185 (90.0531, 12.9607) -> (99.4102, 12.9607)
  line L186 (99.4102, 12.9607) -> (99.4102, 9.8536)
  line L187 (99.4102, 9.8536) -> (95.7674, 9.8536)
  line L188 (95.7674, 9.8536) -> (95.7674, 5.8536)
  line L189 (95.7674, 5.8536) -> (99.4102, 5.8536)
  line L190 (99.4102, 5.8536) -> (99.4102, 2.7464)
  line L191 (93.6959, 9.8536) -> (90.3102, 9.8536)
  line L192 (90.3102, 9.8536) -> (90.3102, 8.4321)
  line L193 (90.3102, 8.4321) -> (88.4888, 8.4321)
  line L194 (88.4888, 8.4321) -> (88.4888, 7.275)
  line L195 (88.4888, 7.275) -> (90.3102, 7.275)
  line L196 (90.3102, 7.275) -> (90.3102, 5.8536)
  line L197 (90.3102, 5.8536) -> (93.6959, 5.8536)
  line L198 (93.6959, 5.8536) -> (93.6959, 9.8536)
  line L199 (99.4102, 15.775) -> (97.5888, 15.775)
  line L200 (97.5888, 15.775) -> (97.5888, 14.3536)
  line L201 (97.5888, 14.3536) -> (88.2317, 14.3536)
  line L202 (88.2317, 14.3536) -> (88.2317, 15.775)
  line L203 (88.2317, 15.775) -> (86.4102, 15.775)
  line L204 (86.4102, 15.775) -> (86.4102, 23.1464)
  line L205 (86.4102, 23.1464) -> (88.2317, 23.1464)
  line L206 (88.2317, 23.1464) -> (88.2317, 24.5679)
  line L207 (88.2317, 24.5679) -> (90.3102, 24.5679)
  line L208 (90.3102, 24.5679) -> (90.3102, 21.4607)
  line L209 (90.3102, 21.4607) -> (88.4888, 21.4607)
  line L210 (88.4888, 21.4607) -> (88.4888, 17.4607)
  line L211 (88.4888, 17.4607) -> (97.3317, 17.4607)
  line L212 (97.3317, 17.4607) -> (97.3317, 21.4607)
  line L213 (97.3317, 21.4607) -> (93.9531, 21.4607)
  line L214 (93.9531, 21.4607) -> (93.9531, 18.6179)
  line L215 (93.9531, 18.6179) -> (91.8745, 18.6179)
  line L216 (91.8745, 18.6179) -> (91.8745, 24.5679)
  line L217 (91.8745, 24.5679) -> (97.5888, 24.5679)
  line L218 (97.5888, 24.5679) -> (97.5888, 23.1464)
  line L219 (97.5888, 23.1464) -> (99.4102, 23.1464)
  line L220 (99.4102, 23.1464) -> (99.4102, 15.775)
  line L221 (99.4102, 27.3821) -> (97.5888, 27.3821)
  line L222 (97.5888, 27.3821) -> (97.5888, 25.9607)
  line L223 (97.5888, 25.9607) -> (88.2317, 25.9607)
  line L224 (88.2317, 25.9607) -> (88.2317, 27.3821)
  line L225 (88.2317, 27.3821) -> (86.4102, 27.3821)
  line L226 (86.4102, 27.3821) -> (86.4102, 34.7536)
  line L227 (86.4102, 34.7536) -> (88.2317, 34.7536)
  line L228 (88.2317, 34.7536) -> (88.2317, 36.175)
  line L229 (88.2317, 36.175) -> (97.5888, 36.175)
  line L230 (97.5888, 36.175) -> (97.5888, 34.7536)
  line L231 (97.5888, 34.7536) -> (99.4102, 34.7536)
  line L232 (99.4102, 34.7536) -> (99.4102, 27.3821)
  line L233 (97.3317, 33.0679) -> (88.4888, 33.0679)
  line L234 (88.4888, 33.0679) -> (88.4888, 29.0679)
  line L235 (88.4888, 29.0679) -> (97.3317, 29.0679)
  line L236 (97.3317, 29.0679) -> (97.3317, 33.0679)
  line L237 (99.4102, 44.675) -> (95.7674, 44.675)
  line L238 (95.7674, 44.675) -> (95.7674, 43.2536)
  line L239 (95.7674, 43.2536) -> (93.6959, 43.2536)
  line L240 (93.6959, 43.2536) -> (93.6959, 44.675)
  line L241 (93.6959, 44.675) -> (86.4102, 44.675)
  line L242 (86.4102, 44.675) -> (86.4102, 47.7821)
  line L243 (86.4102, 47.7821) -> (99.4102, 47.7821)
  line L244 (99.4102, 47.7821) -> (99.4102, 44.675)
  line L245 (99.4102, 37.5679) -> (86.4102, 37.5679)
  line L246 (86.4102, 37.5679) -> (86.4102, 39.2536)
  line L247 (86.4102, 39.2536) -> (88.2317, 39.2536)
  line L248 (88.2317, 39.2536) -> (88.2317, 40.675)
  line L249 (88.2317, 40.675) -> (90.0531, 40.675)
  line L250 (90.0531, 40.675) -> (90.0531, 42.0964)
  line L251 (90.0531, 42.0964) -> (92.1317, 42.0964)
  line L252 (92.1317, 42.0964) -> (92.1317, 40.675)
  line L253 (92.1317, 40.675) -> (99.4102, 40.675)
  line L254 (99.4102, 40.675) -> (99.4102, 37.5679)
  line L255 (93.9531, 41.8321) -> (91.8745, 41.8321)
  line L256 (91.8745, 41.8321) -> (91.8745, 43.5179)
  line L257 (91.8745, 43.5179) -> (93.9531, 43.5179)
  line L258 (93.9531, 43.5179) -> (93.9531, 41.8321)
  point P0 (50.5, 0)
  dimension "d188" = 3
  dimension "d189" = 2
  dimension "d190" = 0
  constraints: 1 point on line, 2 other
  measures "d188" distance between parallel lines of L24 L31
  measures "d189" distance between parallel lines of L18 L29
  measures "d190" distance between parallel lines of L1 L30
extrude "Extrusion4" cut sketch "Sketch5" against normal blind 1 contours L60 L59 L58 L57 L56 L62 L32 | L44 L43 L42 L41 L40 L39 L38 L37 L36 L35 L34 L33 | L55 L54 L53 L52 L51 L50 | L80 L79 L78 L77 L76 L75 L74 L73 | L88 L87 L86 L85 | L102 L101 L100 L99 L98 L97 L96 L95 L94 L93 L92 L91 L90 L89 | L116 L115 L114 L113 L112 L111 L110 L109 L108 L107 | L124 L123 L122 L121 L120 L119 L118 L117 | L128 L127 L126 L125 | L129 L130 L131 L132 L133 L134 L135 L136 | L141 L142 L143 L144 L145 L146 L147 L148 L149 L150 L151 L152 | L157 L158 L159 L160 L161 L162 L163 L164 L165 L166 L167 L168 L169 L170 | L175 L176 L177 L178 L179 L180 L181 L182 L183 L184 L185 L186 L187 L188 L189 L190 | L199 L200 L201 L202 L203 L204 L205 L206 L207 L208 L209 L210 L211 L212 L213 L214 L215 L216 L217 L218 L219 L220 | L221 L222 L223 L224 L225 L226 L227 L228 L229 L230 L231 L232 | L237 L238 L239 L258 L257 L240 L241 L242 L243 L244 | L258 L255 L252 L251 L256 L257 L240 L239 | L239 L240 L257 L258 | L255 L256 L251 L252 | L252 L253 L254 L245 L246 L247 L248 L249 L250 L251 L256 L255
body "Solid2"
